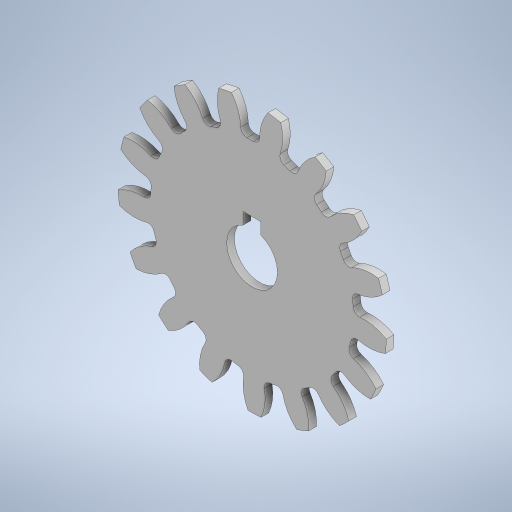
# Autodesk Inventor part: engranaje1
Saved by Autodesk Inventor 2023 (Build 270158000, 158)
## iProperties
Created: 2022-04-26
Part Number: engranaje1
Material: Genérico
Document SubType Name: Modeling
Designer: isaac
Density: 1 g/cm^3
Appearance: Valor por defecto
Author: isaac
Autodesk Inventor part; units mm, degrees
ref_plane "YZ Plane" through (0, 0, 0) normal (1, 0, 0) x (0, 1, 0)
ref_plane "XZ Plane" through (0, 0, 0) normal (0, 1, 0) x (-1, 0, 0)
ref_plane "XY Plane" through (0, 0, 0) normal (0, 0, 1) x (1, 0, 0)
sketch "Boceto1" plane through (0, 0, 0) normal (0, 0, 1) x (1, 0, 0)
  arc A0 (52.913, -1.3839) -> (39.9966, 0.519) centre (44.1511, -16.0697) ccw
  arc A1 (39.4761, -6.4527) -> (52.5319, -6.489) centre (46.0479, 9.3351) ccw
  arc A2 (52.5319, -6.489) -> (52.913, -1.3839) centre (0, 0) ccw
  arc A3 (49.8398, 17.824) -> (37.1083, 14.9324) centre (46.9747, 0.9647) ccw
  arc A4 (39.1414, 8.2434) -> (51.3286, 12.9258) centre (39.5662, 25.3391) ccw
  arc A5 (51.3286, 12.9258) -> (49.8398, 17.824) centre (0, 0) ccw
  arc A6 (40.0355, 34.6246) -> (29.2082, 27.3291) centre (43.4541, 17.8688) ccw
  arc A7 (33.5204, 21.8262) -> (43.1932, 30.595) centre (27.7408, 37.921) ccw
  arc A8 (43.1932, 30.595) -> (40.0355, 34.6246) centre (0, 0) ccw
  arc A9 (24.8242, 46.749) -> (17.3634, 36.0349) centre (34.0648, 32.3596) ccw
  arc A10 (23.3723, 32.4613) -> (29.2242, 44.1322) centre (12.1689, 45.3814) ccw
  arc A11 (29.2242, 44.1322) -> (24.8242, 46.749) centre (0, 0) ccw
  arc A12 (6.2602, 52.5596) -> (3.1736, 39.8739) centre (20.0749, 42.48) ccw
  arc A13 (10.0676, 38.7123) -> (11.3084, 51.709) centre (-5.0465, 46.7128) ccw
  arc A14 (11.3084, 51.709) -> (6.2602, 52.5596) centre (0, 0) ccw
  arc A15 (-13.1493, 51.2718) -> (-11.4448, 38.3278) centre (3.3737, 46.8634) ccw
  arc A16 (-4.5967, 39.735) -> (-8.1347, 52.3023) centre (-21.5803, 41.7354) ccw
  arc A17 (-8.1347, 52.3023) -> (-13.1493, 51.2718) centre (0, 0) ccw
  arc A18 (-30.7829, 43.0595) -> (-24.5175, 31.6052) centre (-13.7831, 44.9175) ccw
  arc A19 (-18.6403, 35.3913) -> (-26.4791, 45.8318) centre (-35.1996, 31.1214) ccw
  arc A20 (-26.4791, 45.8318) -> (-30.7829, 43.0595) centre (0, 0) ccw
  arc A21 (-44.259, 29.0317) -> (-34.279, 20.6142) centre (-29.0784, 36.9053) ccw
  arc A22 (-30.1663, 26.2677) -> (-41.2474, 33.1716) centre (-44.065, 16.3043) ccw
  arc A23 (-41.2474, 33.1716) -> (-44.259, 29.0317) centre (0, 0) ccw
  arc A24 (-51.7578, 11.083) -> (-39.411, 6.8392) centre (-40.4466, 23.9088) ccw
  arc A25 (-37.6183, 13.5966) -> (-50.445, 16.0313) centre (-46.9792, -0.7149) ccw
  arc A26 (-50.445, 16.0313) -> (-51.7578, 11.083) centre (0, 0) ccw
  arc A27 (-52.2664, -8.3624) -> (-39.2202, -7.8595) centre (-46.3522, 7.6833) ccw
  arc A28 (-39.9896, -0.9108) -> (-52.8298, -3.2741) centre (-43.5486, -17.6374) ccw
  arc A29 (-52.8298, -3.2741) -> (-52.2664, -8.3624) centre (0, 0) ccw
  arc A30 (-45.7161, -26.6785) -> (-33.7326, -21.4968) centre (-45.9976, -9.5798) ccw
  arc A31 (-36.9602, -15.2953) -> (-48.0795, -22.1374) centre (-34.2365, -32.178) ccw
  arc A32 (-48.0795, -22.1374) -> (-45.7161, -26.6785) centre (0, 0) ccw
  arc A33 (-32.9916, -41.3915) -> (-23.6892, -32.2308) centre (-39.4309, -25.5492) ccw
  arc A34 (-28.9391, -27.614) -> (-36.8359, -38.0108) centre (-20.3005, -42.3727) ccw
  arc A35 (-36.8359, -38.0108) -> (-32.9916, -41.3915) centre (0, 0) ccw
  arc A36 (-15.8114, -50.5144) -> (-10.4464, -38.6118) centre (-27.5388, -38.068) ccw
  arc A37 (-17.0096, -36.2032) -> (-20.6174, -48.7507) centre (-3.6229, -46.8447) ccw
  arc A38 (-20.6174, -48.7507) -> (-15.8114, -50.5144) centre (0, 0) ccw
  arc A39 (3.5042, -52.815) -> (4.2072, -39.7781) centre (-11.9274, -45.4455) ccw
  arc A40 (-2.7828, -39.9031) -> (-1.6143, -52.9065) centre (13.544, -44.9902) ccw
  arc A41 (-1.6143, -52.9065) -> (3.5042, -52.815) centre (0, 0) ccw
  arc A42 (22.3466, -47.9826) -> (18.2926, -35.5722) centre (5.2948, -46.6853) ccw
  arc A43 (11.8198, -38.2138) -> (17.6067, -49.917) centre (28.8818, -37.0594) ccw
  arc A44 (17.6067, -49.917) -> (22.3466, -47.9826) centre (0, 0) ccw
  arc A45 (38.1709, -36.67) -> (29.9075, -26.562) centre (21.802, -41.6201) ccw
  arc A46 (24.826, -31.3635) -> (34.4499, -40.1859) centre (40.3188, -24.1236) ccw
  arc A47 (34.4499, -40.1859) -> (38.1709, -36.67) centre (0, 0) ccw
  arc A48 (48.84, -20.4048) -> (37.4832, -13.9645) centre (35.3646, -30.9338) ccw
  arc A49 (34.4794, -20.2774) -> (46.6404, -25.0276) centre (46.3106, -7.9297) ccw
  arc A50 (46.6404, -25.0276) -> (48.84, -20.4048) centre (0, 0) ccw
  arc A51 (-11.4448, 38.3278) -> (-18.6403, 35.3913) centre (0, 0) ccw
  arc A52 (-24.5175, 31.6052) -> (-30.1663, 26.2677) centre (0, 0) ccw
  arc A53 (-34.279, 20.6142) -> (-37.6183, 13.5966) centre (0, 0) ccw
  arc A54 (-39.411, 6.8392) -> (-39.9896, -0.9108) centre (0, 0) ccw
  arc A55 (-39.2202, -7.8595) -> (-36.9602, -15.2953) centre (0, 0) ccw
  arc A56 (-33.7326, -21.4968) -> (-28.9391, -27.614) centre (0, 0) ccw
  arc A57 (-23.6892, -32.2308) -> (-17.0096, -36.2032) centre (0, 0) ccw
  arc A58 (-10.4464, -38.6118) -> (-2.7828, -39.9031) centre (0, 0) ccw
  arc A59 (4.2072, -39.7781) -> (11.8198, -38.2138) centre (0, 0) ccw
  arc A60 (18.2926, -35.5722) -> (24.826, -31.3635) centre (0, 0) ccw
  arc A61 (29.9075, -26.562) -> (34.4794, -20.2774) centre (0, 0) ccw
  arc A62 (37.4832, -13.9645) -> (39.4761, -6.4527) centre (0, 0) ccw
  arc A63 (39.9966, 0.519) -> (39.1414, 8.2434) centre (0, 0) ccw
  arc A64 (37.1083, 14.9324) -> (33.5204, 21.8262) centre (0, 0) ccw
  arc A65 (29.2082, 27.3291) -> (23.3723, 32.4613) centre (0, 0) ccw
  arc A66 (17.3634, 36.0349) -> (10.0676, 38.7123) centre (0, 0) ccw
  arc A67 (3.1736, 39.8739) -> (-4.5967, 39.735) centre (0, 0) ccw
  point P0 (59.9974, -0.5572)
  dimension "d8" = 360
  constraints: 136 point on circle, 68 centre point, 36 coincident, 203 other
extrude "Extrusión1" add sketch "Boceto1" along normal blind 3
fillet "Empalme1" radius 2.4 2 edges at (10.0676, 38.7123, 1.5) (17.3634, 36.0349, 1.5)
pattern_circular "Patrón circular1" count 17 over 360 about axis through (0, 0, 0) along (0, 0, 1) of "Empalme1"
sketch "Boceto2" plane through (0, 0, 3) normal (0, 0, 1) x (1, 0, 0)
  arc A0 (-3.5, 9.3675) -> (3.5, 9.3675) centre (0, 0) ccw
  line L0 (3.5, 9.3675) -> (3.5, 14)
  line L1 (3.5, 14) -> (-3.5, 14)
  line L2 (-3.5, 14) -> (-3.5, 9.3675)
  line L3 (2.4254, 9.7014) -> (3.5, 14) construction
  line L4 (-2.4254, 9.7014) -> (-3.5, 14) construction
  point P0 (3.5, 11.6837)
  dimension "d16" = 20
  dimension "d17" = 7
  dimension "d18" = 14
  dimension "d19" = 7
  dimension "d20" = 3.5
  dimension "d21" = 3.5
  constraints: 10 end point, 2 point on circle, 1 centre point, 1 coincident, 1 midpoint, 1 parallel
  measures "d16" diameter of A0
  measures "d17" distance of L1.end L0.end
  measures "d18" distance from line of L1 point (0, 0)
  measures "d19" distance from line of point (3.5, 11.684) L2
  measures "d20" horizontal distance of point (0, 0) L0.end
  measures "d21" horizontal distance of point (0, 0) L2.end
extrude "Extrusión2" cut sketch "Boceto2" against normal blind 3
